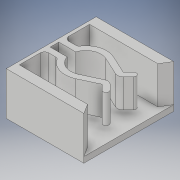
# Autodesk Inventor part: shaft holder clip
Saved by Autodesk Inventor 2019.3 (Build 233278000, 278)
## iProperties
Created: 2018-12-19
Part Number: shaft holder clip
Material: Generic
Document SubType Name: Modeling
Designer: Frienddo
Density: 1 g/cm^3
Appearance: Default
Author: Frienddo
Autodesk Inventor part; units mm, degrees
ref_plane "YZ Plane" through (0, 0, 0) normal (1, 0, 0) x (0, 1, 0)
ref_plane "XZ Plane" through (0, 0, 0) normal (0, 1, 0) x (-1, 0, 0)
ref_plane "XY Plane" through (0, 0, 0) normal (0, 0, 1) x (1, 0, 0)
sketch "Sketch1" plane through (0, 0, 0) normal (0, 1, 0) x (-1, 0, 0)
  circle A0 centre (0, 0) radius 5
  arc A1 (5.25, 0) -> (-2.2187, -4.7581) centre (0, 0) ccw
  line L0 (-2.2187, -4.7581) -> (-8.4373, -1.8583)
  arc A2 (-8.4373, -1.8583) -> (-10.6939, -2.2562) centre (-9.2815, -3.6687) ccw
  line L1 (-10.6939, -2.2562) -> (-12.463, -4.0253)
  arc A3 (-12.463, -4.0253) -> (-11.0487, -5.4395) centre (-11.7558, -4.7324) ccw
  line L2 (-11.0487, -5.4395) -> (-9.281, -3.6717)
  line L3 (-9.281, -3.6717) -> (-3.064, -6.5707)
  arc A4 (-3.064, -6.5707) -> (6.0765, -3.9545) centre (0, 0) ccw
  line L4 (6.9147, -3.5) -> (9.4384, -3.5)
  line L5 (5.0312, -1.5) -> (10.9225, -1.5)
  line L6 (10.9384, -5) -> (10.9384, -12.2255)
  line L7 (10.9384, -12.2255) -> (-12.8, -12.2255)
  line L8 (10.9225, -1.5) -> (10.9225, 0)
  line L9 (12.0588, 0) -> (12.0588, -15.6375)
  line L10 (12.0588, -15.6375) -> (-14.9211, -15.6375)
  line L11 (0, 0) -> (7.7398, 0) construction
  line L12 (-12.8, -12.2255) -> (-14.9211, -15.6375)
  line L13 (10.9225, 0) -> (12.0588, 0)
  arc A5 (5.0312, -1.5) -> (5.25, 0) centre (0, 0) ccw
  arc A6 (-2.2187, -4.7581) -> (5.0312, -1.5) centre (0, 0) ccw
  arc A7 (10.9384, -5) -> (9.4384, -3.5) centre (9.4384, -5) ccw
  arc A8 (6.9147, -3.5) -> (6.0765, -3.9545) centre (6.9147, -4.5) ccw
  line L14 (-2.2187, 4.7581) -> (-8.4373, 1.8583)
  arc A9 (-10.6939, 2.2562) -> (-8.4373, 1.8583) centre (-9.2815, 3.6687) ccw
  line L15 (-10.6939, 2.2562) -> (-12.463, 4.0253)
  arc A10 (-11.0487, 5.4395) -> (-12.463, 4.0253) centre (-11.7558, 4.7324) ccw
  line L16 (-11.0487, 5.4395) -> (-9.281, 3.6717)
  line L17 (-9.281, 3.6717) -> (-3.064, 6.5707)
  arc A11 (6.0765, 3.9545) -> (-3.064, 6.5707) centre (0, 0) ccw
  line L18 (6.9147, 3.5) -> (9.4384, 3.5)
  line L19 (5.0312, 1.5) -> (10.9225, 1.5)
  line L20 (10.9384, 5) -> (10.9384, 12.2255)
  line L21 (10.9384, 12.2255) -> (-12.8, 12.2255)
  line L22 (10.9225, 1.5) -> (10.9225, 0)
  line L23 (12.0588, 0) -> (12.0588, 15.6375)
  line L24 (12.0588, 15.6375) -> (-14.9211, 15.6375)
  line L25 (-12.8, 12.2255) -> (-14.9211, 15.6375)
  arc A12 (5.0312, 1.5) -> (-2.2187, 4.7581) centre (0, 0) ccw
  arc A13 (9.4384, 3.5) -> (10.9384, 5) centre (9.4384, 5) ccw
  arc A14 (6.0765, 3.9545) -> (6.9147, 3.5) centre (6.9147, 4.5) ccw
  point P0 (6.3492, -3.5)
  point P1 (10.9384, -3.5)
  point P2 (6.3492, 3.5)
  point P3 (10.9384, 3.5)
  dimension "d0" = 10
  dimension "d1" = 10.5
  dimension "d2" = 2
  dimension "d3" = 2
  dimension "d4" = 2
  dimension "d5" = 25
  dimension "d6" = 1.5
  dimension "d7" = 110
  dimension "d8" = 2.5
  dimension "d11" = 1.5
  dimension "d12" = 1
  constraints: 52 end point, 30 point on circle, 23 symmetric about line, 15 centre point, 11 tangent, 7 point on line, 3 coincident, 3 horizontal, 3 parallel, 3 vertical, 2 perpendicular, 6 other
  measures "d0" diameter of A0
  measures "d1" diameter of A1
  measures "d2" distance between parallel lines of L5 L4
  measures "d3" radial gap between concentric circles of A1 A4
  measures "d4" distance between parallel lines of L2 L1
  measures "d5" angle of L11 L0
  measures "d6" distance between parallel lines of L11 L5
  measures "d7" angle of L3 L2
  measures "d8" distance of L2.start L2.end
  measures "d11" radius of A7
  measures "d12" radius of A8
extrude "Extrusion1" add sketch "Sketch1" along normal blind 10 contours A1 L14 A9 L15 A10 L16 L17 A11 A14 L18 A13 L20 L21 L25 L24 L23 L13 L22 L19 | L5 L8 L13 L9 L10 L12 L7 L6 A7 L4 A8 A4 L3 L2 A3 L1 A2 L0 A6
sketch "Sketch2" plane through (0, 0, 0) normal (0, -1, 0) x (1, 0, 0)
  line L0 (-10.9225, 1.5) -> (-10.9225, -1.5) projected
  line L1 (-5.0312, 1.5) -> (-10.9225, 1.5) projected
  arc A0 (2.2187, 4.7581) -> (-5.0312, 1.5) centre (0, 0) ccw projected
  line L2 (8.4373, 1.8583) -> (2.2187, 4.7581) projected
  arc A1 (8.4373, 1.8583) -> (10.6939, 2.2562) centre (9.2815, 3.6687) ccw projected
  line L3 (12.463, 4.0253) -> (10.6939, 2.2562) projected
  arc A2 (12.463, 4.0253) -> (11.0487, 5.4395) centre (11.7558, 4.7324) ccw projected
  line L4 (9.281, 3.6717) -> (11.0487, 5.4395) projected
  line L5 (3.064, 6.5707) -> (9.281, 3.6717) projected
  arc A3 (3.064, 6.5707) -> (-6.0765, 3.9545) centre (0, 0) ccw projected
  arc A4 (-6.9147, 3.5) -> (-6.0765, 3.9545) centre (-6.9147, 4.5) ccw projected
  line L6 (-9.4384, 3.5) -> (-6.9147, 3.5) projected
  arc A5 (-10.9384, 5) -> (-9.4384, 3.5) centre (-9.4384, 5) ccw projected
  line L7 (-10.9384, 12.2255) -> (-10.9384, 5) projected
  line L8 (12.8, 12.2255) -> (-10.9384, 12.2255) projected
  line L9 (14.9211, 15.6375) -> (12.8, 12.2255) projected
  line L10 (-12.0588, 15.6375) -> (14.9211, 15.6375) projected
  line L11 (-12.0588, -15.6375) -> (-12.0588, 15.6375) projected
  line L12 (14.9211, -15.6375) -> (-12.0588, -15.6375) projected
  line L13 (12.8, -12.2255) -> (14.9211, -15.6375) projected
  line L14 (-10.9384, -12.2255) -> (12.8, -12.2255) projected
  line L15 (-10.9384, -5) -> (-10.9384, -12.2255) projected
  arc A6 (-9.4384, -3.5) -> (-10.9384, -5) centre (-9.4384, -5) ccw projected
  line L16 (-6.9147, -3.5) -> (-9.4384, -3.5) projected
  arc A7 (-6.0765, -3.9545) -> (-6.9147, -3.5) centre (-6.9147, -4.5) ccw projected
  arc A8 (-6.0765, -3.9545) -> (3.064, -6.5707) centre (0, 0) ccw projected
  line L17 (9.281, -3.6717) -> (3.064, -6.5707) projected
  line L18 (11.0487, -5.4395) -> (9.281, -3.6717) projected
  arc A9 (11.0487, -5.4395) -> (12.463, -4.0253) centre (11.7558, -4.7324) ccw projected
  line L19 (10.6939, -2.2562) -> (12.463, -4.0253) projected
  arc A10 (10.6939, -2.2562) -> (8.4373, -1.8583) centre (9.2815, -3.6687) ccw projected
  line L20 (2.2187, -4.7581) -> (8.4373, -1.8583) projected
  arc A11 (-5.0312, -1.5) -> (2.2187, -4.7581) centre (0, 0) ccw projected
  line L21 (-10.9225, -1.5) -> (-5.0312, -1.5) projected
  arc A12 (-9.4384, -3.5) -> (-10.9384, -5) centre (-9.4384, -5) ccw projected
  line L22 (-10.9384, 5) -> (-10.9384, -5)
  constraints: 2 end point, 1 tangent, 1 vertical
extrude "Extrusion2" add sketch "Sketch2" along normal blind 3 contours L22 L15 L14 L13 L12 L11 L10 L9 L8 L7
sketch "Sketch3" plane through (0, -3, 0) normal (0, -1, 0) x (1, 0, 0)
  line L0 (14.9211, -15.6375) -> (12.8, -12.2255) projected
  line L1 (-12.0588, 15.6375) -> (14.9211, 15.6375)
  line L2 (14.9211, 15.6375) -> (14.9211, -15.6375)
  line L3 (14.9211, -15.6375) -> (-12.0588, -15.6375)
  line L4 (-12.0588, -15.6375) -> (-12.0588, 15.6375)
  point P0 (0, 0)
  constraints: 8 end point, 2 parallel, 1 horizontal, 1 perpendicular
extrude "Extrusion3" add sketch "Sketch3" along normal blind 2
body "Solid1"
